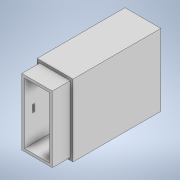
# Autodesk Inventor part: obudowa_latarka
Saved by Autodesk Inventor 2020.4 (Build 244396000, 396)
## iProperties
Created: 2021-06-08
Part Number: obudowa_latarka
Material: Ogólny
Document SubType Name: Modeling
Designer: przem
Density: 1 g/cm^3
Appearance: Domyślna
Author: przem
Autodesk Inventor part; units mm, degrees
ref_plane "YZ Plane" through (0, 0, 0) normal (1, 0, 0) x (0, 1, 0)
ref_plane "XZ Plane" through (0, 0, 0) normal (0, 1, 0) x (-1, 0, 0)
ref_plane "XY Plane" through (0, 0, 0) normal (0, 0, 1) x (1, 0, 0)
sketch "Szkic1" plane through (0, 0, 0) normal (0, 0, 1) x (1, 0, 0)
  line L0 (0, 0) -> (20, 0)
  line L1 (20, 0) -> (20, 40)
  line L2 (20, 40) -> (0, 40)
  line L3 (0, 40) -> (0, 0)
  circle A0 centre (10, 20) radius 3
  dimension "d0" = 20
  dimension "d1" = 40
  dimension "d2" = 6
  constraints: 8 end point, 2 parallel, 1 centre point, 1 horizontal, 1 perpendicular
  measures "d0" distance of L2.end L1.end
  measures "d1" distance of L1.end L0.end
  measures "d2" diameter of A0
extrude "Wyciągnięcie proste1" add sketch "Szkic1" along normal blind 49
sketch "Szkic2" plane through (0, 0, 49) normal (0, 0, 1) x (1, 0, 0)
  line L0 (3, 37) -> (17, 37)
  line L1 (17, 37) -> (17, 3)
  line L2 (17, 3) -> (3, 3)
  line L3 (3, 3) -> (3, 37)
  line L4 (0, 0) -> (20, 0) projected
  line L5 (20, 40) -> (0, 40) projected
  line L6 (0, 40) -> (0, 0) projected
  line L7 (20, 0) -> (20, 40) projected
  dimension "d5" = 14
  dimension "d6" = 34
  dimension "d7" = 3
  dimension "d8" = 3
  dimension "d9" = 3
  dimension "d10" = 3
  constraints: 8 end point, 2 parallel, 1 horizontal, 1 perpendicular
  measures "d5" distance of L1.end L2.end
  measures "d6" distance of L0.end L1.end
  measures "d7" distance between parallel lines of L4 L2
  measures "d8" distance between parallel lines of L5 L0
  measures "d9" distance between parallel lines of L6 L3
  measures "d10" distance between parallel lines of L7 L1
extrude "Wyciągnięcie proste2" cut sketch "Szkic2" against normal blind 46 contours L0 L1 L2 L3
sketch "Szkic3" plane through (0, 0, 49) normal (0, 0, 1) x (1, 0, 0)
  line L0 (3, 3) -> (3, 37) projected
  line L1 (3, 37) -> (17, 37) projected
  line L2 (3, 3) -> (17, 3)
  line L3 (17, 3) -> (17, 37)
  line L4 (17, 37) -> (3, 37)
  line L5 (3, 37) -> (3, 3)
  line L6 (17, 3) -> (3, 3) construction
  line L7 (3, 3) -> (3, 1.5) construction
  line L8 (3, 1.5) -> (1.5, 1.5) construction
  line L9 (1.5, 1.5) -> (18.5, 1.5)
  line L10 (18.5, 1.5) -> (18.5, 38.5)
  line L11 (18.5, 38.5) -> (1.5, 38.5)
  line L12 (1.5, 38.5) -> (1.5, 1.5)
  point P0 (0, 0)
  dimension "d13" = 1.5
  dimension "d14" = 1.5
  dimension "d15" = 34
  dimension "d16" = 14
  dimension "d17" = 17
  dimension "d18" = 37
  constraints: 20 end point, 4 parallel, 3 perpendicular, 2 horizontal, 1 point on line
  measures "d13" distance of L0.start L7.end
  measures "d14" distance of L7.end L8.end
  measures "d15" distance of L0.start L0.end
  measures "d16" distance of L0.start L2.end
  measures "d17" distance of L11.end L10.end
  measures "d18" distance of L10.end L9.end
extrude "Wyciągnięcie proste3" add sketch "Szkic3" along normal blind 10
sketch "Szkic4" plane through (0, 0, 0) normal (-1, 0, 0) x (0, 0, 1)
  line L0 (0, 0) -> (0, 20)
  line L1 (0, 0) -> (0, 40) projected
  line L2 (0, 20) -> (16.8, 20)
  circle A0 centre (16.8, 20) radius 10
  dimension "d21" = 16.8
  dimension "d22" = 20
  constraints: 4 end point, 1 centre point, 1 coincident, 1 midpoint, 1 perpendicular
  measures "d21" distance of L0.end L2.end
  measures "d22" diameter of A0
extrude "Wyciągnięcie proste4" cut sketch "Szkic4" against normal up to surface (3 mm away)
sketch "Szkic5" plane through (1.5, 1.5, 49) normal (-1, 0, 0) x (0, 0, 1)
  line L0 (0, 0) -> (10, 0) construction
  line L1 (0, 37) -> (10, 37) construction
  line L2 (10, 0) -> (0, 37) construction
  line L3 (0, 37) -> (10, 37) construction
  line L4 (10, 37) -> (0, 0) construction
  line L5 (0, 38.5) -> (0, -1.5) construction
  line L6 (5.5, 20.5) -> (4.5, 20.5)
  line L7 (4.5, 20.5) -> (4.5, 16.5)
  line L8 (4.5, 16.5) -> (5.5, 16.5)
  line L9 (5.5, 16.5) -> (5.5, 20.5)
  line L10 (5.5, 20.5) -> (4.5, 16.5) construction
  line L11 (4.5, 20.5) -> (5.5, 16.5) construction
  point P0 (-49, -1.5)
  point P1 (5, 18.5)
  dimension "d25" = 1
  dimension "d26" = 4
  constraints: 18 end point, 3 equal length, 3 midpoint, 1 horizontal, 1 perpendicular, 1 point on line
  measures "d25" distance of L8.end L7.end
  measures "d26" distance of L7.end L6.end
extrude "Wyciągnięcie proste5" cut sketch "Szkic5" against normal up to surface (1.5 mm away)
equation "\"d7\" = d8"
equation "\"d9\" = d10"
equation "\"d14\" = d13"
equation "\"d17\" = d16 + 2 * d14"
equation "\"d18\" = d15 + 2 * d14"
